Autodesk Fusion 360 part; units mm, degrees
(part 2 of 2)
  spline S12 degree 5 poles (2.837383, 13.23075) (2.840225, 13.244003) (2.8454, 13.270575) (2.851636, 13.310634) (2.857051, 13.364425) (2.859891, 13.432189) (2.859938, 13.500337) (2.858297, 13.56873) (2.855743, 13.637265) (2.852533, 13.705893) (2.848599, 13.774606) (2.843687, 13.843415) (2.837503, 13.912339) (2.829877, 13.981384) (2.820834, 14.05054) (2.810501, 14.119787) (2.799061, 14.189099) (2.786693, 14.258453) (2.773501, 14.327831) (2.75951, 14.397224) (2.744699, 14.46663) (2.729023, 14.536047) (2.712438, 14.605473) (2.694933, 14.674904) (2.676527, 14.744334) (2.657255, 14.813755) (2.637157, 14.883156) (2.616273, 14.952531) (2.594626, 15.021871) (2.572224, 15.091173) (2.54907, 15.160431) (2.525161, 15.229641) (2.500496, 15.298799) (2.475081, 15.367901) (2.448924, 15.436941) (2.422038, 15.505915) (2.394436, 15.574817) (2.36613, 15.643643) (2.337129, 15.712387) (2.30744, 15.781046) (2.277067, 15.849615) (2.246015, 15.91809) (2.214289, 15.986467) (2.181892, 16.054742) (2.148832, 16.122912) (2.115115, 16.190971) (2.080748, 16.258916) (2.045735, 16.326743) (2.010083, 16.394449) (1.973797, 16.462029) (1.936882, 16.529479) (1.899341, 16.596797) (1.861179, 16.663979) (1.8224, 16.73102) (1.783009, 16.797918) (1.743011, 16.864669) (1.70241, 16.931268) (1.661209, 16.997713) (1.619414, 17.064) (1.577028, 17.130127) (1.534055, 17.196091) (1.490498, 17.261887) (1.446361, 17.327515) (1.401648, 17.392968) (1.356364, 17.458244) (1.310511, 17.523339) (1.264095, 17.588249) (1.217118, 17.652969) (1.169585, 17.717499) (1.121497, 17.781836) (1.072858, 17.845981) (1.033505, 17.897141) (1.003743, 17.935424) (0.983792, 17.960908) (0.973788, 17.97364) knots 0 0 0 0 0 0 0.01428571 0.02857143 0.04285714 0.05714286 0.07142857 0.08571429 0.1 0.11428571 0.12857143 0.14285714 0.15714286 0.17142857 0.18571429 0.2 0.21428571 0.22857143 0.24285714 0.25714286 0.27142857 0.28571429 0.3 0.31428571 0.32857143 0.34285714 0.35714286 0.37142857 0.38571429 0.4 0.41428571 0.42857143 0.44285714 0.45714286 0.47142857 0.48571429 0.5 0.51428571 0.52857143 0.54285714 0.55714286 0.57142857 0.58571429 0.6 0.61428571 0.62857143 0.64285714 0.65714286 0.67142857 0.68571429 0.7 0.71428571 0.72857143 0.74285714 0.75714286 0.77142857 0.78571429 0.8 0.81428571 0.82857143 0.84285714 0.85714286 0.87142857 0.88571429 0.9 0.91428571 0.92857143 0.94285714 0.95714286 0.97142857 0.98571429 1 1 1 1 1 1
  arc A26 (0.973788, 17.97364) -> (-0.973788, 17.97364) centre (0, 0) ccw
  spline S13 degree 5 poles (-0.973788, 17.97364) (-0.983792, 17.960908) (-1.003743, 17.935424) (-1.033505, 17.897141) (-1.072858, 17.845981) (-1.121497, 17.781836) (-1.169585, 17.717499) (-1.217118, 17.652969) (-1.264095, 17.588249) (-1.310511, 17.523339) (-1.356364, 17.458244) (-1.401648, 17.392968) (-1.446361, 17.327515) (-1.490498, 17.261887) (-1.534055, 17.196091) (-1.577028, 17.130127) (-1.619414, 17.064) (-1.661209, 16.997713) (-1.70241, 16.931268) (-1.743011, 16.864669) (-1.783009, 16.797918) (-1.8224, 16.73102) (-1.861179, 16.663979) (-1.899341, 16.596797) (-1.936882, 16.529479) (-1.973797, 16.462029) (-2.010083, 16.394449) (-2.045735, 16.326743) (-2.080748, 16.258916) (-2.115115, 16.190971) (-2.148832, 16.122912) (-2.181892, 16.054742) (-2.214289, 15.986467) (-2.246015, 15.91809) (-2.277067, 15.849615) (-2.30744, 15.781046) (-2.337129, 15.712387) (-2.36613, 15.643643) (-2.394436, 15.574817) (-2.422038, 15.505915) (-2.448924, 15.436941) (-2.475081, 15.367901) (-2.500496, 15.298799) (-2.525161, 15.229641) (-2.54907, 15.160431) (-2.572224, 15.091173) (-2.594626, 15.021871) (-2.616273, 14.952531) (-2.637157, 14.883156) (-2.657255, 14.813755) (-2.676527, 14.744334) (-2.694933, 14.674904) (-2.712438, 14.605473) (-2.729023, 14.536047) (-2.744699, 14.46663) (-2.75951, 14.397224) (-2.773501, 14.327831) (-2.786693, 14.258453) (-2.799061, 14.189099) (-2.810501, 14.119787) (-2.820834, 14.05054) (-2.829877, 13.981384) (-2.837503, 13.912339) (-2.843687, 13.843415) (-2.848599, 13.774606) (-2.852533, 13.705893) (-2.855743, 13.637265) (-2.858297, 13.56873) (-2.859938, 13.500337) (-2.859891, 13.432189) (-2.857051, 13.364425) (-2.851636, 13.310634) (-2.8454, 13.270575) (-2.840225, 13.244003) (-2.837383, 13.23075) knots -1 -1 -1 -1 -1 -1 -0.98571429 -0.97142857 -0.95714286 -0.94285714 -0.92857143 -0.91428571 -0.9 -0.88571429 -0.87142857 -0.85714286 -0.84285714 -0.82857143 -0.81428571 -0.8 -0.78571429 -0.77142857 -0.75714286 -0.74285714 -0.72857143 -0.71428571 -0.7 -0.68571429 -0.67142857 -0.65714286 -0.64285714 -0.62857143 -0.61428571 -0.6 -0.58571429 -0.57142857 -0.55714286 -0.54285714 -0.52857143 -0.51428571 -0.5 -0.48571429 -0.47142857 -0.45714286 -0.44285714 -0.42857143 -0.41428571 -0.4 -0.38571429 -0.37142857 -0.35714286 -0.34285714 -0.32857143 -0.31428571 -0.3 -0.28571429 -0.27142857 -0.25714286 -0.24285714 -0.22857143 -0.21428571 -0.2 -0.18571429 -0.17142857 -0.15714286 -0.14285714 -0.12857143 -0.11428571 -0.1 -0.08571429 -0.07142857 -0.05714286 -0.04285714 -0.02857143 -0.01428571 0 0 0 0 0 0
  line L13 (-2.837383, 13.23075) -> (-2.384479, 11.118854)
  arc A27 (-3.184436, 9.726793) -> (-2.384479, 11.118854) centre (-3.557802, 10.86723) ccw
  arc A28 (-3.184436, 9.726793) -> (-4.626145, 9.129617) centre (0, 0) ccw
  arc A29 (-6.176136, 9.548298) -> (-4.626145, 9.129617) centre (-5.168547, 10.200038) ccw
  line L14 (-6.176136, 9.548298) -> (-7.34922, 11.361886)
  spline S14 degree 5 poles (-7.34922, 11.361886) (-7.356582, 11.373267) (-7.371712, 11.395716) (-7.395628, 11.42845) (-7.429836, 11.470315) (-7.475743, 11.52024) (-7.523898, 11.568461) (-7.57342, 11.615662) (-7.623687, 11.662318) (-7.674485, 11.708575) (-7.725854, 11.754381) (-7.777982, 11.799563) (-7.831092, 11.843926) (-7.885306, 11.887356) (-7.940601, 11.929863) (-7.996873, 11.971521) (-8.053973, 12.012444) (-8.111759, 12.052738) (-8.170145, 12.092468) (-8.229106, 12.131644) (-8.288657, 12.170248) (-8.348827, 12.208248) (-8.409646, 12.245612) (-8.471119, 12.28233) (-8.533228, 12.318409) (-8.595944, 12.353869) (-8.659229, 12.388733) (-8.723051, 12.423021) (-8.78739, 12.456745) (-8.852234, 12.489908) (-8.917579, 12.522508) (-8.983424, 12.554541) (-9.049766, 12.586002) (-9.1166, 12.616893) (-9.183915, 12.647217) (-9.251698, 12.676977) (-9.319937, 12.706181) (-9.38862, 12.734832) (-9.457736, 12.762935) (-9.527279, 12.790491) (-9.597241, 12.8175) (-9.667617, 12.843962) (-9.738401, 12.869878) (-9.809586, 12.895248) (-9.881166, 12.920074) (-9.953133, 12.944358) (-10.025479, 12.968101) (-10.098198, 12.991304) (-10.171282, 13.013969) (-10.244727, 13.036098) (-10.318525, 13.057689) (-10.392671, 13.078745) (-10.46716, 13.099265) (-10.541987, 13.119249) (-10.617144, 13.1387) (-10.692627, 13.157616) (-10.768429, 13.176) (-10.844546, 13.19385) (-10.920971, 13.211169) (-10.997702, 13.227957) (-11.074732, 13.244213) (-11.152056, 13.259939) (-11.229671, 13.275135) (-11.307571, 13.289801) (-11.385749, 13.303937) (-11.464201, 13.317543) (-11.54292, 13.33062) (-11.621902, 13.343167) (-11.701142, 13.355185) (-11.780639, 13.366676) (-11.860389, 13.377639) (-11.924391, 13.385988) (-11.972507, 13.392014) (-12.004634, 13.395926) (-12.02071, 13.397855) knots 0 0 0 0 0 0 0.01428571 0.02857143 0.04285714 0.05714286 0.07142857 0.08571429 0.1 0.11428571 0.12857143 0.14285714 0.15714286 0.17142857 0.18571429 0.2 0.21428571 0.22857143 0.24285714 0.25714286 0.27142857 0.28571429 0.3 0.31428571 0.32857143 0.34285714 0.35714286 0.37142857 0.38571429 0.4 0.41428571 0.42857143 0.44285714 0.45714286 0.47142857 0.48571429 0.5 0.51428571 0.52857143 0.54285714 0.55714286 0.57142857 0.58571429 0.6 0.61428571 0.62857143 0.64285714 0.65714286 0.67142857 0.68571429 0.7 0.71428571 0.72857143 0.74285714 0.75714286 0.77142857 0.78571429 0.8 0.81428571 0.82857143 0.84285714 0.85714286 0.87142857 0.88571429 0.9 0.91428571 0.92857143 0.94285714 0.95714286 0.97142857 0.98571429 1 1 1 1 1 1
  arc A30 (-12.02071, 13.397855) -> (-13.397855, 12.02071) centre (0, 0) ccw
  spline S15 degree 5 poles (-13.397855, 12.02071) (-13.395926, 12.004634) (-13.392014, 11.972507) (-13.385988, 11.924391) (-13.377639, 11.860389) (-13.366676, 11.780639) (-13.355185, 11.701142) (-13.343167, 11.621902) (-13.33062, 11.54292) (-13.317543, 11.464201) (-13.303937, 11.385749) (-13.289801, 11.307571) (-13.275135, 11.229671) (-13.259939, 11.152056) (-13.244213, 11.074732) (-13.227957, 10.997702) (-13.211169, 10.920971) (-13.19385, 10.844546) (-13.176, 10.768429) (-13.157616, 10.692627) (-13.1387, 10.617144) (-13.119249, 10.541987) (-13.099265, 10.46716) (-13.078745, 10.392671) (-13.057689, 10.318525) (-13.036098, 10.244727) (-13.013969, 10.171282) (-12.991304, 10.098198) (-12.968101, 10.025479) (-12.944358, 9.953133) (-12.920074, 9.881166) (-12.895248, 9.809586) (-12.869878, 9.738401) (-12.843962, 9.667617) (-12.8175, 9.597241) (-12.790491, 9.527279) (-12.762935, 9.457736) (-12.734832, 9.38862) (-12.706181, 9.319937) (-12.676977, 9.251698) (-12.647217, 9.183915) (-12.616893, 9.1166) (-12.586002, 9.049766) (-12.554541, 8.983424) (-12.522508, 8.917579) (-12.489908, 8.852234) (-12.456745, 8.78739) (-12.423021, 8.723051) (-12.388733, 8.659229) (-12.353869, 8.595944) (-12.318409, 8.533228) (-12.28233, 8.471119) (-12.245612, 8.409646) (-12.208248, 8.348827) (-12.170248, 8.288657) (-12.131644, 8.229106) (-12.092468, 8.170145) (-12.052738, 8.111759) (-12.012444, 8.053973) (-11.971521, 7.996873) (-11.929863, 7.940601) (-11.887356, 7.885306) (-11.843926, 7.831092) (-11.799563, 7.777982) (-11.754381, 7.725854) (-11.708575, 7.674485) (-11.662318, 7.623687) (-11.615662, 7.57342) (-11.568461, 7.523898) (-11.52024, 7.475743) (-11.470315, 7.429836) (-11.42845, 7.395628) (-11.395716, 7.371712) (-11.373267, 7.356582) (-11.361886, 7.34922) knots -1 -1 -1 -1 -1 -1 -0.98571429 -0.97142857 -0.95714286 -0.94285714 -0.92857143 -0.91428571 -0.9 -0.88571429 -0.87142857 -0.85714286 -0.84285714 -0.82857143 -0.81428571 -0.8 -0.78571429 -0.77142857 -0.75714286 -0.74285714 -0.72857143 -0.71428571 -0.7 -0.68571429 -0.67142857 -0.65714286 -0.64285714 -0.62857143 -0.61428571 -0.6 -0.58571429 -0.57142857 -0.55714286 -0.54285714 -0.52857143 -0.51428571 -0.5 -0.48571429 -0.47142857 -0.45714286 -0.44285714 -0.42857143 -0.41428571 -0.4 -0.38571429 -0.37142857 -0.35714286 -0.34285714 -0.32857143 -0.31428571 -0.3 -0.28571429 -0.27142857 -0.25714286 -0.24285714 -0.22857143 -0.21428571 -0.2 -0.18571429 -0.17142857 -0.15714286 -0.14285714 -0.12857143 -0.11428571 -0.1 -0.08571429 -0.07142857 -0.05714286 -0.04285714 -0.02857143 -0.01428571 0 0 0 0 0 0
  line L15 (-11.361886, 7.34922) -> (-9.548298, 6.176136)
  arc A31 (-9.129617, 4.626145) -> (-9.548298, 6.176136) centre (-10.200038, 5.168547) ccw
  circle A32 centre (0, 0) radius 1.15
  line L16 (3.025234, 9.791883) -> (-3.025234, 9.791883)
  line L17 (3.025234, 9.791883) -> (3.439485, 19.18384)
  line L18 (3.439485, 19.18384) -> (-4.990636, 19.555668)
  line L19 (-4.990636, 19.555668) -> (-3.025234, 9.791883)
  line L20 (-9.854685, -2.913789) -> (-10.545247, 2.401806)
  line L21 (-10.545247, 2.401806) -> (-19, 8)
  line L22 (-19, 8) -> (-21.442412, -5.346157)
  line L23 (-21.442412, -5.346157) -> (-9.854685, -2.913789)
  line L24 (2.770942, -9.961222) -> (-2.770942, -9.961222)
  line L25 (-2.770942, -9.961222) -> (-5.656102, -20.555719)
  line L26 (-5.656102, -20.555719) -> (4.796523, -17.724881)
  line L27 (4.796523, -17.724881) -> (2.770942, -9.961222)
  line L28 (9.947362, -2.78719) -> (10.269334, 2.51736)
  line L29 (10.269334, 2.51736) -> (19.086106, 5.71213)
  line L30 (19.086106, 5.71213) -> (21.537563, -1.953993)
  line L31 (21.537563, -1.953993) -> (14.67772, -5.231594)
  line L32 (14.67772, -5.231594) -> (9.947362, -2.78719)
  constraint horizontal L16
  constraint perpendicular L17 L18
  constraint horizontal L24
extrude "Extrude3" cut sketch "Sketch1" against normal blind 2 contours A1 L0 S0 A2 S1 L1 A3 L20 | A25 L12 S12 A26 S13 L13 A27 L16 | A9 L4 S4 A10 S5 L5 A11 L24 | A17 L8 S8 A18 S9 L9 A19 L28 picked at (-12.526785, 0.794826) picked at (-0.794826, 12.526785) picked at (0.794826, -12.526785) picked at (12.526785, -0.794826) bodies 2 in component "Spur Gear 8 teeth (1)"
combine "Combine1" operation add target body 1 tool bodies 2 in component "Spur Gear 8 teeth"
sketch "Sketch2" plane through (0, 0, 6.5) normal (0, 0, 1) x (-1, 0, 0)
  line L0 (9.947362, -2.78719) -> (10.269334, 2.51736)
  arc A0 (9.726793, 3.184436) -> (10.269334, 2.51736) centre (10.86723, 3.557802) ccw
  arc A1 (9.726793, 3.184436) -> (9.129617, 4.626145) centre (0, 0) ccw
  arc A2 (9.548298, 6.176136) -> (9.129617, 4.626145) centre (10.200038, 5.168547) ccw
  line L1 (9.548298, 6.176136) -> (11.361886, 7.34922)
  spline S0 degree 5 poles (11.361886, 7.34922) (11.373267, 7.356582) (11.395716, 7.371712) (11.42845, 7.395628) (11.470315, 7.429836) (11.52024, 7.475743) (11.568461, 7.523898) (11.615662, 7.57342) (11.662318, 7.623687) (11.708575, 7.674485) (11.754381, 7.725854) (11.799563, 7.777982) (11.843926, 7.831092) (11.887356, 7.885306) (11.929863, 7.940601) (11.971521, 7.996873) (12.012444, 8.053973) (12.052738, 8.111759) (12.092468, 8.170145) (12.131644, 8.229106) (12.170248, 8.288657) (12.208248, 8.348827) (12.245612, 8.409646) (12.28233, 8.471119) (12.318409, 8.533228) (12.353869, 8.595944) (12.388733, 8.659229) (12.423021, 8.723051) (12.456745, 8.78739) (12.489908, 8.852234) (12.522508, 8.917579) (12.554541, 8.983424) (12.586002, 9.049766) (12.616893, 9.1166) (12.647217, 9.183915) (12.676977, 9.251698) (12.706181, 9.319937) (12.734832, 9.38862) (12.762935, 9.457736) (12.790491, 9.527279) (12.8175, 9.597241) (12.843962, 9.667617) (12.869878, 9.738401) (12.895248, 9.809586) (12.920074, 9.881166) (12.944358, 9.953133) (12.968101, 10.025479) (12.991304, 10.098198) (13.013969, 10.171282) (13.036098, 10.244727) (13.057689, 10.318525) (13.078745, 10.392671) (13.099265, 10.46716) (13.119249, 10.541987) (13.1387, 10.617144) (13.157616, 10.692627) (13.176, 10.768429) (13.19385, 10.844546) (13.211169, 10.920971) (13.227957, 10.997702) (13.244213, 11.074732) (13.259939, 11.152056) (13.275135, 11.229671) (13.289801, 11.307571) (13.303937, 11.385749) (13.317543, 11.464201) (13.33062, 11.54292) (13.343167, 11.621902) (13.355185, 11.701142) (13.366676, 11.780639) (13.377639, 11.860389) (13.385988, 11.924391) (13.392014, 11.972507) (13.395926, 12.004634) (13.397855, 12.02071) knots 0 0 0 0 0 0 0.01428571 0.02857143 0.04285714 0.05714286 0.07142857 0.08571429 0.1 0.11428571 0.12857143 0.14285714 0.15714286 0.17142857 0.18571429 0.2 0.21428571 0.22857143 0.24285714 0.25714286 0.27142857 0.28571429 0.3 0.31428571 0.32857143 0.34285714 0.35714286 0.37142857 0.38571429 0.4 0.41428571 0.42857143 0.44285714 0.45714286 0.47142857 0.48571429 0.5 0.51428571 0.52857143 0.54285714 0.55714286 0.57142857 0.58571429 0.6 0.61428571 0.62857143 0.64285714 0.65714286 0.67142857 0.68571429 0.7 0.71428571 0.72857143 0.74285714 0.75714286 0.77142857 0.78571429 0.8 0.81428571 0.82857143 0.84285714 0.85714286 0.87142857 0.88571429 0.9 0.91428571 0.92857143 0.94285714 0.95714286 0.97142857 0.98571429 1 1 1 1 1 1
  arc A3 (13.397855, 12.02071) -> (12.02071, 13.397855) centre (0, 0) ccw
  spline S1 degree 5 poles (12.02071, 13.397855) (12.004634, 13.395926) (11.972507, 13.392014) (11.924391, 13.385988) (11.860389, 13.377639) (11.780639, 13.366676) (11.701142, 13.355185) (11.621902, 13.343167) (11.54292, 13.33062) (11.464201, 13.317543) (11.385749, 13.303937) (11.307571, 13.289801) (11.229671, 13.275135) (11.152056, 13.259939) (11.074732, 13.244213) (10.997702, 13.227957) (10.920971, 13.211169) (10.844546, 13.19385) (10.768429, 13.176) (10.692627, 13.157616) (10.617144, 13.1387) (10.541987, 13.119249) (10.46716, 13.099265) (10.392671, 13.078745) (10.318525, 13.057689) (10.244727, 13.036098) (10.171282, 13.013969) (10.098198, 12.991304) (10.025479, 12.968101) (9.953133, 12.944358) (9.881166, 12.920074) (9.809586, 12.895248) (9.738401, 12.869878) (9.667617, 12.843962) (9.597241, 12.8175) (9.527279, 12.790491) (9.457736, 12.762935) (9.38862, 12.734832) (9.319937, 12.706181) (9.251698, 12.676977) (9.183915, 12.647217) (9.1166, 12.616893) (9.049766, 12.586002) (8.983424, 12.554541) (8.917579, 12.522508) (8.852234, 12.489908) (8.78739, 12.456745) (8.723051, 12.423021) (8.659229, 12.388733) (8.595944, 12.353869) (8.533228, 12.318409) (8.471119, 12.28233) (8.409646, 12.245612) (8.348827, 12.208248) (8.288657, 12.170248) (8.229106, 12.131644) (8.170145, 12.092468) (8.111759, 12.052738) (8.053973, 12.012444) (7.996873, 11.971521) (7.940601, 11.929863) (7.885306, 11.887356) (7.831092, 11.843926) (7.777982, 11.799563) (7.725854, 11.754381) (7.674485, 11.708575) (7.623687, 11.662318) (7.57342, 11.615662) (7.523898, 11.568461) (7.475743, 11.52024) (7.429836, 11.470315) (7.395628, 11.42845) (7.371712, 11.395716) (7.356582, 11.373267) (7.34922, 11.361886) knots -1 -1 -1 -1 -1 -1 -0.98571429 -0.97142857 -0.95714286 -0.94285714 -0.92857143 -0.91428571 -0.9 -0.88571429 -0.87142857 -0.85714286 -0.84285714 -0.82857143 -0.81428571 -0.8 -0.78571429 -0.77142857 -0.75714286 -0.74285714 -0.72857143 -0.71428571 -0.7 -0.68571429 -0.67142857 -0.65714286 -0.64285714 -0.62857143 -0.61428571 -0.6 -0.58571429 -0.57142857 -0.55714286 -0.54285714 -0.52857143 -0.51428571 -0.5 -0.48571429 -0.47142857 -0.45714286 -0.44285714 -0.42857143 -0.41428571 -0.4 -0.38571429 -0.37142857 -0.35714286 -0.34285714 -0.32857143 -0.31428571 -0.3 -0.28571429 -0.27142857 -0.25714286 -0.24285714 -0.22857143 -0.21428571 -0.2 -0.18571429 -0.17142857 -0.15714286 -0.14285714 -0.12857143 -0.11428571 -0.1 -0.08571429 -0.07142857 -0.05714286 -0.04285714 -0.02857143 -0.01428571 0 0 0 0 0 0
  line L2 (7.34922, 11.361886) -> (6.176136, 9.548298)
  arc A4 (4.626145, 9.129617) -> (6.176136, 9.548298) centre (5.168547, 10.200038) ccw
  arc A5 (4.626145, 9.129617) -> (3.184436, 9.726793) centre (0, 0) ccw
  arc A6 (3.025234, 9.791883) -> (3.184436, 9.726793) centre (3.557802, 10.86723) ccw
  line L3 (3.025234, 9.791883) -> (-3.025234, 9.791883)
  arc A7 (-3.184436, 9.726793) -> (-3.025234, 9.791883) centre (-3.557802, 10.86723) ccw
  arc A8 (-3.184436, 9.726793) -> (-4.626145, 9.129617) centre (0, 0) ccw
  arc A9 (-6.176136, 9.548298) -> (-4.626145, 9.129617) centre (-5.168547, 10.200038) ccw
  line L4 (-6.176136, 9.548298) -> (-7.34922, 11.361886)
  spline S2 degree 5 poles (-7.34922, 11.361886) (-7.356582, 11.373267) (-7.371712, 11.395716) (-7.395628, 11.42845) (-7.429836, 11.470315) (-7.475743, 11.52024) (-7.523898, 11.568461) (-7.57342, 11.615662) (-7.623687, 11.662318) (-7.674485, 11.708575) (-7.725854, 11.754381) (-7.777982, 11.799563) (-7.831092, 11.843926) (-7.885306, 11.887356) (-7.940601, 11.929863) (-7.996873, 11.971521) (-8.053973, 12.012444) (-8.111759, 12.052738) (-8.170145, 12.092468) (-8.229106, 12.131644) (-8.288657, 12.170248) (-8.348827, 12.208248) (-8.409646, 12.245612) (-8.471119, 12.28233) (-8.533228, 12.318409) (-8.595944, 12.353869) (-8.659229, 12.388733) (-8.723051, 12.423021) (-8.78739, 12.456745) (-8.852234, 12.489908) (-8.917579, 12.522508) (-8.983424, 12.554541) (-9.049766, 12.586002) (-9.1166, 12.616893) (-9.183915, 12.647217) (-9.251698, 12.676977) (-9.319937, 12.706181) (-9.38862, 12.734832) (-9.457736, 12.762935) (-9.527279, 12.790491) (-9.597241, 12.8175) (-9.667617, 12.843962) (-9.738401, 12.869878) (-9.809586, 12.895248) (-9.881166, 12.920074) (-9.953133, 12.944358) (-10.025479, 12.968101) (-10.098198, 12.991304) (-10.171282, 13.013969) (-10.244727, 13.036098) (-10.318525, 13.057689) (-10.392671, 13.078745) (-10.46716, 13.099265) (-10.541987, 13.119249) (-10.617144, 13.1387) (-10.692627, 13.157616) (-10.768429, 13.176) (-10.844546, 13.19385) (-10.920971, 13.211169) (-10.997702, 13.227957) (-11.074732, 13.244213) (-11.152056, 13.259939) (-11.229671, 13.275135) (-11.307571, 13.289801) (-11.385749, 13.303937) (-11.464201, 13.317543) (-11.54292, 13.33062) (-11.621902, 13.343167) (-11.701142, 13.355185) (-11.780639, 13.366676) (-11.860389, 13.377639) (-11.924391, 13.385988) (-11.972507, 13.392014) (-12.004634, 13.395926) (-12.02071, 13.397855) knots 0 0 0 0 0 0 0.01428571 0.02857143 0.04285714 0.05714286 0.07142857 0.08571429 0.1 0.11428571 0.12857143 0.14285714 0.15714286 0.17142857 0.18571429 0.2 0.21428571 0.22857143 0.24285714 0.25714286 0.27142857 0.28571429 0.3 0.31428571 0.32857143 0.34285714 0.35714286 0.37142857 0.38571429 0.4 0.41428571 0.42857143 0.44285714 0.45714286 0.47142857 0.48571429 0.5 0.51428571 0.52857143 0.54285714 0.55714286 0.57142857 0.58571429 0.6 0.61428571 0.62857143 0.64285714 0.65714286 0.67142857 0.68571429 0.7 0.71428571 0.72857143 0.74285714 0.75714286 0.77142857 0.78571429 0.8 0.81428571 0.82857143 0.84285714 0.85714286 0.87142857 0.88571429 0.9 0.91428571 0.92857143 0.94285714 0.95714286 0.97142857 0.98571429 1 1 1 1 1 1
  arc A10 (-12.02071, 13.397855) -> (-13.397855, 12.02071) centre (0, 0) ccw
  spline S3 degree 5 poles (-13.397855, 12.02071) (-13.395926, 12.004634) (-13.392014, 11.972507) (-13.385988, 11.924391) (-13.377639, 11.860389) (-13.366676, 11.780639) (-13.355185, 11.701142) (-13.343167, 11.621902) (-13.33062, 11.54292) (-13.317543, 11.464201) (-13.303937, 11.385749) (-13.289801, 11.307571) (-13.275135, 11.229671) (-13.259939, 11.152056) (-13.244213, 11.074732) (-13.227957, 10.997702) (-13.211169, 10.920971) (-13.19385, 10.844546) (-13.176, 10.768429) (-13.157616, 10.692627) (-13.1387, 10.617144) (-13.119249, 10.541987) (-13.099265, 10.46716) (-13.078745, 10.392671) (-13.057689, 10.318525) (-13.036098, 10.244727) (-13.013969, 10.171282) (-12.991304, 10.098198) (-12.968101, 10.025479) (-12.944358, 9.953133) (-12.920074, 9.881166) (-12.895248, 9.809586) (-12.869878, 9.738401) (-12.843962, 9.667617) (-12.8175, 9.597241) (-12.790491, 9.527279) (-12.762935, 9.457736) (-12.734832, 9.38862) (-12.706181, 9.319937) (-12.676977, 9.251698) (-12.647217, 9.183915) (-12.616893, 9.1166) (-12.586002, 9.049766) (-12.554541, 8.983424) (-12.522508, 8.917579) (-12.489908, 8.852234) (-12.456745, 8.78739) (-12.423021, 8.723051) (-12.388733, 8.659229) (-12.353869, 8.595944) (-12.318409, 8.533228) (-12.28233, 8.471119) (-12.245612, 8.409646) (-12.208248, 8.348827) (-12.170248, 8.288657) (-12.131644, 8.229106) (-12.092468, 8.170145) (-12.052738, 8.111759) (-12.012444, 8.053973) (-11.971521, 7.996873) (-11.929863, 7.940601) (-11.887356, 7.885306) (-11.843926, 7.831092) (-11.799563, 7.777982) (-11.754381, 7.725854) (-11.708575, 7.674485) (-11.662318, 7.623687) (-11.615662, 7.57342) (-11.568461, 7.523898) (-11.52024, 7.475743) (-11.470315, 7.429836) (-11.42845, 7.395628) (-11.395716, 7.371712) (-11.373267, 7.356582) (-11.361886, 7.34922) knots -1 -1 -1 -1 -1 -1 -0.98571429 -0.97142857 -0.95714286 -0.94285714 -0.92857143 -0.91428571 -0.9 -0.88571429 -0.87142857 -0.85714286 -0.84285714 -0.82857143 -0.81428571 -0.8 -0.78571429 -0.77142857 -0.75714286 -0.74285714 -0.72857143 -0.71428571 -0.7 -0.68571429 -0.67142857 -0.65714286 -0.64285714 -0.62857143 -0.61428571 -0.6 -0.58571429 -0.57142857 -0.55714286 -0.54285714 -0.52857143 -0.51428571 -0.5 -0.48571429 -0.47142857 -0.45714286 -0.44285714 -0.42857143 -0.41428571 -0.4 -0.38571429 -0.37142857 -0.35714286 -0.34285714 -0.32857143 -0.31428571 -0.3 -0.28571429 -0.27142857 -0.25714286 -0.24285714 -0.22857143 -0.21428571 -0.2 -0.18571429 -0.17142857 -0.15714286 -0.14285714 -0.12857143 -0.11428571 -0.1 -0.08571429 -0.07142857 -0.05714286 -0.04285714 -0.02857143 -0.01428571 0 0 0 0 0 0
  line L5 (-11.361886, 7.34922) -> (-9.548298, 6.176136)
  arc A11 (-9.129617, 4.626145) -> (-9.548298, 6.176136) centre (-10.200038, 5.168547) ccw
  arc A12 (-9.129617, 4.626145) -> (-9.726793, 3.184436) centre (0, 0) ccw
  arc A13 (-10.545247, 2.401806) -> (-9.726793, 3.184436) centre (-10.86723, 3.557802) ccw
  line L6 (-10.545247, 2.401806) -> (-9.854685, -2.913789)
  arc A14 (-9.726793, -3.184436) -> (-9.854685, -2.913789) centre (-10.86723, -3.557802) ccw
  arc A15 (-9.726793, -3.184436) -> (-9.129617, -4.626145) centre (0, 0) ccw
  arc A16 (-9.548298, -6.176136) -> (-9.129617, -4.626145) centre (-10.200038, -5.168547) ccw
  line L7 (-9.548298, -6.176136) -> (-11.361886, -7.34922)
  spline S4 degree 5 poles (-11.361886, -7.34922) (-11.373267, -7.356582) (-11.395716, -7.371712) (-11.42845, -7.395628) (-11.470315, -7.429836) (-11.52024, -7.475743) (-11.568461, -7.523898) (-11.615662, -7.57342) (-11.662318, -7.623687) (-11.708575, -7.674485) (-11.754381, -7.725854) (-11.799563, -7.777982) (-11.843926, -7.831092) (-11.887356, -7.885306) (-11.929863, -7.940601) (-11.971521, -7.996873) (-12.012444, -8.053973) (-12.052738, -8.111759) (-12.092468, -8.170145) (-12.131644, -8.229106) (-12.170248, -8.288657) (-12.208248, -8.348827) (-12.245612, -8.409646) (-12.28233, -8.471119) (-12.318409, -8.533228) (-12.353869, -8.595944) (-12.388733, -8.659229) (-12.423021, -8.723051) (-12.456745, -8.78739) (-12.489908, -8.852234) (-12.522508, -8.917579) (-12.554541, -8.983424) (-12.586002, -9.049766) (-12.616893, -9.1166) (-12.647217, -9.183915) (-12.676977, -9.251698) (-12.706181, -9.319937) (-12.734832, -9.38862) (-12.762935, -9.457736) (-12.790491, -9.527279) (-12.8175, -9.597241) (-12.843962, -9.667617) (-12.869878, -9.738401) (-12.895248, -9.809586) (-12.920074, -9.881166) (-12.944358, -9.953133) (-12.968101, -10.025479) (-12.991304, -10.098198) (-13.013969, -10.171282) (-13.036098, -10.244727) (-13.057689, -10.318525) (-13.078745, -10.392671) (-13.099265, -10.46716) (-13.119249, -10.541987) (-13.1387, -10.617144) (-13.157616, -10.692627) (-13.176, -10.768429) (-13.19385, -10.844546) (-13.211169, -10.920971) (-13.227957, -10.997702) (-13.244213, -11.074732) (-13.259939, -11.152056) (-13.275135, -11.229671) (-13.289801, -11.307571) (-13.303937, -11.385749) (-13.317543, -11.464201) (-13.33062, -11.54292) (-13.343167, -11.621902) (-13.355185, -11.701142) (-13.366676, -11.780639) (-13.377639, -11.860389) (-13.385988, -11.924391) (-13.392014, -11.972507) (-13.395926, -12.004634) (-13.397855, -12.02071) knots 0 0 0 0 0 0 0.01428571 0.02857143 0.04285714 0.05714286 0.07142857 0.08571429 0.1 0.11428571 0.12857143 0.14285714 0.15714286 0.17142857 0.18571429 0.2 0.21428571 0.22857143 0.24285714 0.25714286 0.27142857 0.28571429 0.3 0.31428571 0.32857143 0.34285714 0.35714286 0.37142857 0.38571429 0.4 0.41428571 0.42857143 0.44285714 0.45714286 0.47142857 0.48571429 0.5 0.51428571 0.52857143 0.54285714 0.55714286 0.57142857 0.58571429 0.6 0.61428571 0.62857143 0.64285714 0.65714286 0.67142857 0.68571429 0.7 0.71428571 0.72857143 0.74285714 0.75714286 0.77142857 0.78571429 0.8 0.81428571 0.82857143 0.84285714 0.85714286 0.87142857 0.88571429 0.9 0.91428571 0.92857143 0.94285714 0.95714286 0.97142857 0.98571429 1 1 1 1 1 1
  arc A17 (-13.397855, -12.02071) -> (-12.02071, -13.397855) centre (0, 0) ccw
  spline S5 degree 5 poles (-12.02071, -13.397855) (-12.004634, -13.395926) (-11.972507, -13.392014) (-11.924391, -13.385988) (-11.860389, -13.377639) (-11.780639, -13.366676) (-11.701142, -13.355185) (-11.621902, -13.343167) (-11.54292, -13.33062) (-11.464201, -13.317543) (-11.385749, -13.303937) (-11.307571, -13.289801) (-11.229671, -13.275135) (-11.152056, -13.259939) (-11.074732, -13.244213) (-10.997702, -13.227957) (-10.920971, -13.211169) (-10.844546, -13.19385) (-10.768429, -13.176) (-10.692627, -13.157616) (-10.617144, -13.1387) (-10.541987, -13.119249) (-10.46716, -13.099265) (-10.392671, -13.078745) (-10.318525, -13.057689) (-10.244727, -13.036098) (-10.171282, -13.013969) (-10.098198, -12.991304) (-10.025479, -12.968101) (-9.953133, -12.944358) (-9.881166, -12.920074) (-9.809586, -12.895248) (-9.738401, -12.869878) (-9.667617, -12.843962) (-9.597241, -12.8175) (-9.527279, -12.790491) (-9.457736, -12.762935) (-9.38862, -12.734832) (-9.319937, -12.706181) (-9.251698, -12.676977) (-9.183915, -12.647217) (-9.1166, -12.616893) (-9.049766, -12.586002) (-8.983424, -12.554541) (-8.917579, -12.522508) (-8.852234, -12.489908) (-8.78739, -12.456745) (-8.723051, -12.423021) (-8.659229, -12.388733) (-8.595944, -12.353869) (-8.533228, -12.318409) (-8.471119, -12.28233) (-8.409646, -12.245612) (-8.348827, -12.208248) (-8.288657, -12.170248) (-8.229106, -12.131644) (-8.170145, -12.092468) (-8.111759, -12.052738) (-8.053973, -12.012444) (-7.996873, -11.971521) (-7.940601, -11.929863) (-7.885306, -11.887356) (-7.831092, -11.843926) (-7.777982, -11.799563) (-7.725854, -11.754381) (-7.674485, -11.708575) (-7.623687, -11.662318) (-7.57342, -11.615662) (-7.523898, -11.568461) (-7.475743, -11.52024) (-7.429836, -11.470315) (-7.395628, -11.42845) (-7.371712, -11.395716) (-7.356582, -11.373267) (-7.34922, -11.361886) knots -1 -1 -1 -1 -1 -1 -0.98571429 -0.97142857 -0.95714286 -0.94285714 -0.92857143 -0.91428571 -0.9 -0.88571429 -0.87142857 -0.85714286 -0.84285714 -0.82857143 -0.81428571 -0.8 -0.78571429 -0.77142857 -0.75714286 -0.74285714 -0.72857143 -0.71428571 -0.7 -0.68571429 -0.67142857 -0.65714286 -0.64285714 -0.62857143 -0.61428571 -0.6 -0.58571429 -0.57142857 -0.55714286 -0.54285714 -0.52857143 -0.51428571 -0.5 -0.48571429 -0.47142857 -0.45714286 -0.44285714 -0.42857143 -0.41428571 -0.4 -0.38571429 -0.37142857 -0.35714286 -0.34285714 -0.32857143 -0.31428571 -0.3 -0.28571429 -0.27142857 -0.25714286 -0.24285714 -0.22857143 -0.21428571 -0.2 -0.18571429 -0.17142857 -0.15714286 -0.14285714 -0.12857143 -0.11428571 -0.1 -0.08571429 -0.07142857 -0.05714286 -0.04285714 -0.02857143 -0.01428571 0 0 0 0 0 0
  line L8 (-7.34922, -11.361886) -> (-6.176136, -9.548298)
  arc A18 (-4.626145, -9.129617) -> (-6.176136, -9.548298) centre (-5.168547, -10.200038) ccw
  arc A19 (-4.626145, -9.129617) -> (-3.184436, -9.726793) centre (0, 0) ccw
  arc A20 (-2.770942, -9.961222) -> (-3.184436, -9.726793) centre (-3.557802, -10.86723) ccw
  line L9 (-2.770942, -9.961222) -> (2.770942, -9.961222)
  arc A21 (3.184436, -9.726793) -> (2.770942, -9.961222) centre (3.557802, -10.86723) ccw
  arc A22 (3.184436, -9.726793) -> (4.626145, -9.129617) centre (0, 0) ccw
  arc A23 (6.176136, -9.548298) -> (4.626145, -9.129617) centre (5.168547, -10.200038) ccw
  line L10 (6.176136, -9.548298) -> (7.34922, -11.361886)
  spline S6 degree 5 poles (7.34922, -11.361886) (7.356582, -11.373267) (7.371712, -11.395716) (7.395628, -11.42845) (7.429836, -11.470315) (7.475743, -11.52024) (7.523898, -11.568461) (7.57342, -11.615662) (7.623687, -11.662318) (7.674485, -11.708575) (7.725854, -11.754381) (7.777982, -11.799563) (7.831092, -11.843926) (7.885306, -11.887356) (7.940601, -11.929863) (7.996873, -11.971521) (8.053973, -12.012444) (8.111759, -12.052738) (8.170145, -12.092468) (8.229106, -12.131644) (8.288657, -12.170248) (8.348827, -12.208248) (8.409646, -12.245612) (8.471119, -12.28233) (8.533228, -12.318409) (8.595944, -12.353869) (8.659229, -12.388733) (8.723051, -12.423021) (8.78739, -12.456745) (8.852234, -12.489908) (8.917579, -12.522508) (8.983424, -12.554541) (9.049766, -12.586002) (9.1166, -12.616893) (9.183915, -12.647217) (9.251698, -12.676977) (9.319937, -12.706181) (9.38862, -12.734832) (9.457736, -12.762935) (9.527279, -12.790491) (9.597241, -12.8175) (9.667617, -12.843962) (9.738401, -12.869878) (9.809586, -12.895248) (9.881166, -12.920074) (9.953133, -12.944358) (10.025479, -12.968101) (10.098198, -12.991304) (10.171282, -13.013969) (10.244727, -13.036098) (10.318525, -13.057689) (10.392671, -13.078745) (10.46716, -13.099265) (10.541987, -13.119249) (10.617144, -13.1387) (10.692627, -13.157616) (10.768429, -13.176) (10.844546, -13.19385) (10.920971, -13.211169) (10.997702, -13.227957) (11.074732, -13.244213) (11.152056, -13.259939) (11.229671, -13.275135) (11.307571, -13.289801) (11.385749, -13.303937) (11.464201, -13.317543) (11.54292, -13.33062) (11.621902, -13.343167) (11.701142, -13.355185) (11.780639, -13.366676) (11.860389, -13.377639) (11.924391, -13.385988) (11.972507, -13.392014) (12.004634, -13.395926) (12.02071, -13.397855) knots 0 0 0 0 0 0 0.01428571 0.02857143 0.04285714 0.05714286 0.07142857 0.08571429 0.1 0.11428571 0.12857143 0.14285714 0.15714286 0.17142857 0.18571429 0.2 0.21428571 0.22857143 0.24285714 0.25714286 0.27142857 0.28571429 0.3 0.31428571 0.32857143 0.34285714 0.35714286 0.37142857 0.38571429 0.4 0.41428571 0.42857143 0.44285714 0.45714286 0.47142857 0.48571429 0.5 0.51428571 0.52857143 0.54285714 0.55714286 0.57142857 0.58571429 0.6 0.61428571 0.62857143 0.64285714 0.65714286 0.67142857 0.68571429 0.7 0.71428571 0.72857143 0.74285714 0.75714286 0.77142857 0.78571429 0.8 0.81428571 0.82857143 0.84285714 0.85714286 0.87142857 0.88571429 0.9 0.91428571 0.92857143 0.94285714 0.95714286 0.97142857 0.98571429 1 1 1 1 1 1
  arc A24 (12.02071, -13.397855) -> (13.397855, -12.02071) centre (0, 0) ccw
  spline S7 degree 5 poles (13.397855, -12.02071) (13.395926, -12.004634) (13.392014, -11.972507) (13.385988, -11.924391) (13.377639, -11.860389) (13.366676, -11.780639) (13.355185, -11.701142) (13.343167, -11.621902) (13.33062, -11.54292) (13.317543, -11.464201) (13.303937, -11.385749) (13.289801, -11.307571) (13.275135, -11.229671) (13.259939, -11.152056) (13.244213, -11.074732) (13.227957, -10.997702) (13.211169, -10.920971) (13.19385, -10.844546) (13.176, -10.768429) (13.157616, -10.692627) (13.1387, -10.617144) (13.119249, -10.541987) (13.099265, -10.46716) (13.078745, -10.392671) (13.057689, -10.318525) (13.036098, -10.244727) (13.013969, -10.171282) (12.991304, -10.098198) (12.968101, -10.025479) (12.944358, -9.953133) (12.920074, -9.881166) (12.895248, -9.809586) (12.869878, -9.738401) (12.843962, -9.667617) (12.8175, -9.597241) (12.790491, -9.527279) (12.762935, -9.457736) (12.734832, -9.38862) (12.706181, -9.319937) (12.676977, -9.251698) (12.647217, -9.183915) (12.616893, -9.1166) (12.586002, -9.049766) (12.554541, -8.983424) (12.522508, -8.917579) (12.489908, -8.852234) (12.456745, -8.78739) (12.423021, -8.723051) (12.388733, -8.659229) (12.353869, -8.595944) (12.318409, -8.533228) (12.28233, -8.471119) (12.245612, -8.409646) (12.208248, -8.348827) (12.170248, -8.288657) (12.131644, -8.229106) (12.092468, -8.170145) (12.052738, -8.111759) (12.012444, -8.053973) (11.971521, -7.996873) (11.929863, -7.940601) (11.887356, -7.885306) (11.843926, -7.831092) (11.799563, -7.777982) (11.754381, -7.725854) (11.708575, -7.674485) (11.662318, -7.623687) (11.615662, -7.57342) (11.568461, -7.523898) (11.52024, -7.475743) (11.470315, -7.429836) (11.42845, -7.395628) (11.395716, -7.371712) (11.373267, -7.356582) (11.361886, -7.34922) knots -1 -1 -1 -1 -1 -1 -0.98571429 -0.97142857 -0.95714286 -0.94285714 -0.92857143 -0.91428571 -0.9 -0.88571429 -0.87142857 -0.85714286 -0.84285714 -0.82857143 -0.81428571 -0.8 -0.78571429 -0.77142857 -0.75714286 -0.74285714 -0.72857143 -0.71428571 -0.7 -0.68571429 -0.67142857 -0.65714286 -0.64285714 -0.62857143 -0.61428571 -0.6 -0.58571429 -0.57142857 -0.55714286 -0.54285714 -0.52857143 -0.51428571 -0.5 -0.48571429 -0.47142857 -0.45714286 -0.44285714 -0.42857143 -0.41428571 -0.4 -0.38571429 -0.37142857 -0.35714286 -0.34285714 -0.32857143 -0.31428571 -0.3 -0.28571429 -0.27142857 -0.25714286 -0.24285714 -0.22857143 -0.21428571 -0.2 -0.18571429 -0.17142857 -0.15714286 -0.14285714 -0.12857143 -0.11428571 -0.1 -0.08571429 -0.07142857 -0.05714286 -0.04285714 -0.02857143 -0.01428571 0 0 0 0 0 0
  line L11 (11.361886, -7.34922) -> (9.548298, -6.176136)
  arc A25 (9.129617, -4.626145) -> (9.548298, -6.176136) centre (10.200038, -5.168547) ccw
  arc A26 (9.129617, -4.626145) -> (9.726793, -3.184436) centre (0, 0) ccw
  arc A27 (9.947362, -2.78719) -> (9.726793, -3.184436) centre (10.86723, -3.557802) ccw
  circle A28 centre (0, 0) radius 1.15
  circle A29 centre (0, 0) radius 1.15
  circle A30 centre (0, 0) radius 2.25
  dimension "d19" = 4.5
  constraint concentric A1 A29
  constraint coincident A1.centre A3.centre
  measures "d19" diameter of A30
extrude "Extrude3'" add sketch "Sketch2" along normal blind 12 contours A30 picked at (1.870675, -0.168915) bodies 1 in component "Spur Gear 8 teeth"
chamfer "Chamfer1" distance 0.5 angle 45 1 faces at (0.028647, -6.971145, 0) on bodies 1 in component "Spur Gear 8 teeth"
chamfer "Chamfer2" distance 0.3 angle 45 1 faces at (0.056048, -7.275825, 6.5) on bodies 1 in component "Spur Gear 8 teeth"
chamfer "Chamfer3" distance 0.2 angle 45 1 faces at (-1.870675, 0.168915, 18.5) on bodies 1 in component "Spur Gear 8 teeth"
component "Spur Gear 8 teeth (1)" placed x (1, 0, 0) y (0, 1, 0) z (0, 0, 1) at (0, 0, 0)
component "Spur Gear 8 teeth" placed x (1, 0, 0) y (0, 1, 0) z (0, 0, 1) at (0, 0, 0)
